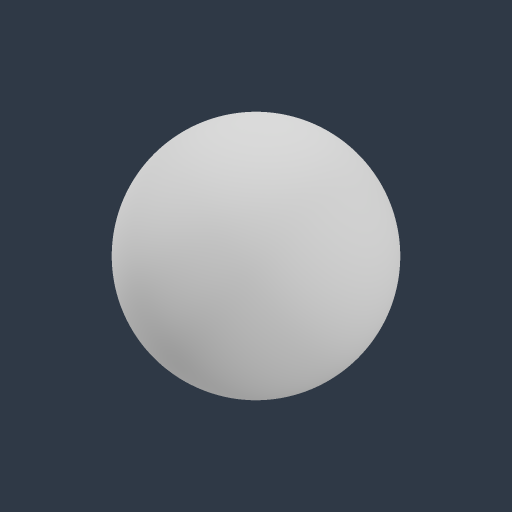
# Autodesk Inventor part: algae
Saved by Autodesk Inventor 2024.3 (Build 283343000, 343)
## iProperties
Created: 2025-02-05
Part Number: algae
Material: Generic
Document SubType Name: Modeling
Designer: Marcus Tannini
Density: 1 g/cm^3
Appearance: Default
Author: Marcus Tannini
Autodesk Inventor part; units mm, degrees
ref_plane "YZ Plane" through (0, 0, 0) normal (1, 0, 0) x (0, 1, 0)
ref_plane "XZ Plane" through (0, 0, 0) normal (0, 1, 0) x (-1, 0, 0)
ref_plane "XY Plane" through (0, 0, 0) normal (0, 0, 1) x (1, 0, 0)
sketch "Sketch1" plane through (0, 0, 0) normal (0, 1, 0) x (-1, 0, 0)
  arc A0 (203.2, 0) -> (-203.2, 0) centre (0, 0) ccw
  line L0 (203.2, 0) -> (-203.2, 0)
  line L1 (284.48, 0) -> (-284.48, 0) projected
  dimension "d0" = 406.4
  dimension "d1" = 406.4
  constraints: 2 end point, 2 point on circle, 1 centre point, 1 coincident, 1 horizontal
  measures "d0" diameter of A0
  measures "d1" distance of L0.start L0.end
revolve "Revolution1" add sketch "Sketch1" angle 360 about axis through (-10, 0, 0) along (1, 0, 0)
equation "\"d1\" = d0"
body "Solid1"
